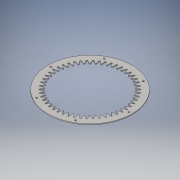
# Autodesk Inventor part: Arm Outer Gear
Saved by Autodesk Inventor 2016 (Build 200138000, 138)
## iProperties
Created: 2016-04-16
Part Number: Arm Outer Gear
Material: Generic
Document SubType Name: Modeling
Designer: rmarkowi
Density: 1 g/cm^3
Appearance: Default
Author: rmarkowi
Autodesk Inventor part; units mm, degrees
(part 1 of 2)
ref_plane "YZ Plane" through (0, 0, 0) normal (1, 0, 0) x (0, 1, 0)
ref_plane "XZ Plane" through (0, 0, 0) normal (0, 1, 0) x (-1, 0, 0)
ref_plane "XY Plane" through (0, 0, 0) normal (0, 0, 1) x (1, 0, 0)
sketch "Sketch1" plane through (0, 0, 0) normal (0, 1, 0) x (-1, 0, 0)
  circle A0 centre (0, 0) radius 120.65 construction
  line L0 (0, 0) -> (120.65, 0) construction
  line L1 (120.65, 120.65) -> (120.65, -120.65) construction
  line L2 (79.3853, 113.3739) -> (161.9147, -113.3739) construction
  line L3 (106.5438, 38.7788) -> (0, 0) construction
  arc A1 (106.5438, 38.7788) -> (102.7586, 47.9171) centre (0, 0) ccw construction
  line L4 (0, 0) -> (102.7586, 47.9171) construction
  line L5 (0, 0) -> (106.5438, 38.7788) construction
  line L6 (102.7586, 47.9171) -> (126.968, 2.8527) construction
  arc A2 (110.9039, 23.5734) -> (106.5438, 38.7788) centre (0, 0) ccw construction
  line L7 (0, 0) -> (110.9039, 23.5734) construction
  line L8 (0, 0) -> (106.5438, 38.7788) construction
  line L9 (110.9039, 23.5734) -> (116.206, -1.371) construction
  line L10 (115.9739, -1.4203) -> (113.3644, -1.975) construction
  spline S0 degree 3 poles (125.457, 2.1829) (119.9346, -0.2189) (115.9739, -1.4203) (113.3644, -1.975) knots 1.081688 1.081688 1.081688 1.081688 2 2 2 2
  line L11 (0, 0) -> (153.1146, 4.8118) construction
  line L12 (0, 0) -> (153.1902, 0) construction
  line L13 (0, 0) -> (153.1146, -4.8118) construction
  line L14 (115.8342, -5.8646) -> (113.2647, -5.1471) construction
  spline S1 degree 3 poles (125.0724, -10.0561) (119.7117, -7.3123) (115.8342, -5.8646) (113.2647, -5.1471) knots 1.081688 1.081688 1.081688 1.081688 2 2 2 2
  circle A3 centre (0, 0) radius 125.476 construction
  line L15 (125.457, 2.1829) -> (119.9346, -0.2189) construction
  line L16 (119.9346, -0.2189) -> (115.9739, -1.4203) construction
  line L17 (125.0724, -10.0561) -> (119.7117, -7.3123) construction
  line L18 (119.7117, -7.3123) -> (115.8342, -5.8646) construction
  arc A4 (126.6012, -10.0561) -> (126.9812, 2.1829) centre (0, 0) ccw
  arc A5 (113.2647, -5.1471) -> (113.3644, -1.975) centre (0, 0) ccw
  line L19 (125.457, 2.1829) -> (126.9812, 2.1829)
  line L20 (125.0724, -10.0561) -> (126.6012, -10.0561)
  arc A6 (113.0167, 9.0893) -> (112.718, 12.2489) centre (0, 0) ccw
  line L21 (115.6558, 8.6996) -> (113.0167, 9.0893) construction
  spline S2 degree 3 poles (124.1942, 17.8896) (119.0164, 14.8147) (115.2374, 13.1263) (112.718, 12.2489) knots 1.081688 1.081688 1.081688 1.081688 2 2 2 2
  line L22 (124.1942, 17.8896) -> (119.0164, 14.8147) construction
  line L23 (119.0164, 14.8147) -> (115.2374, 13.1263) construction
  line L24 (115.2374, 13.1263) -> (112.718, 12.2489) construction
  spline S3 degree 3 poles (125.3465, 5.6989) (119.6842, 7.7492) (115.6558, 8.6996) (113.0167, 9.0893) knots 1.081688 1.081688 1.081688 1.081688 2 2 2 2
  line L25 (125.3465, 5.6989) -> (119.6842, 7.7492) construction
  line L26 (119.6842, 7.7492) -> (115.6558, 8.6996) construction
  arc A7 (126.8633, 5.8906) -> (125.7064, 18.0806) centre (0, 0) ccw
  line L27 (125.3465, 5.6989) -> (126.8633, 5.8906)
  line L28 (124.1942, 17.8896) -> (125.7064, 18.0806)
  arc A8 (110.9863, 23.1824) -> (110.294, 26.2796) centre (0, 0) ccw
  line L29 (113.6535, 23.1265) -> (110.9863, 23.1824) construction
  spline S4 degree 3 poles (120.9727, 33.3142) (116.2211, 29.6145) (112.6836, 27.4658) (110.294, 26.2796) knots 1.081688 1.081688 1.081688 1.081688 2 2 2 2
  line L30 (120.9727, 33.3142) -> (116.2211, 29.6145) construction
  line L31 (116.2211, 29.6145) -> (112.6836, 27.4658) construction
  line L32 (112.6836, 27.4658) -> (110.294, 26.2796) construction
  spline S5 degree 3 poles (123.6439, 21.3641) (117.7693, 22.6885) (113.6535, 23.1265) (110.9863, 23.1824) knots 1.081688 1.081688 1.081688 1.081688 2 2 2 2
  line L33 (123.6439, 21.3641) -> (117.7693, 22.6885) construction
  line L34 (117.7693, 22.6885) -> (113.6535, 23.1265) construction
  arc A9 (125.1247, 21.7443) -> (122.449, 33.6932) centre (0, 0) ccw
  line L35 (123.6439, 21.3641) -> (125.1247, 21.7443)
  line L36 (120.9727, 33.3142) -> (122.449, 33.6932)
  arc A10 (107.2056, 36.9098) -> (106.1306, 39.8959) centre (0, 0) ccw
  line L37 (109.8588, 37.1887) -> (107.2056, 36.9098) construction
  spline S6 degree 3 poles (115.8434, 48.2134) (111.593, 43.9474) (108.3526, 41.3723) (106.1306, 39.8959) knots 1.081688 1.081688 1.081688 1.081688 2 2 2 2
  line L38 (115.8434, 48.2134) -> (111.593, 43.9474) construction
  line L39 (111.593, 43.9474) -> (108.3526, 41.3723) construction
  line L40 (108.3526, 41.3723) -> (106.1306, 39.8959) construction
  spline S7 degree 3 poles (119.9913, 36.6923) (113.997, 37.27) (109.8588, 37.1887) (107.2056, 36.9098) knots 1.081688 1.081688 1.081688 1.081688 2 2 2 2
  line L41 (119.9913, 36.6923) -> (113.997, 37.27) construction
  line L42 (113.997, 37.27) -> (109.8588, 37.1887) construction
  arc A11 (121.4127, 37.2551) -> (117.2606, 48.7745) centre (0, 0) ccw
  line L43 (119.9913, 36.6923) -> (121.4127, 37.2551)
  line L44 (115.8434, 48.2134) -> (117.2606, 48.7745)
  arc A12 (101.7343, 50.0552) -> (100.2934, 52.883) centre (0, 0) ccw
  line L45 (104.3316, 50.6644) -> (101.7343, 50.0552) construction
  spline S8 degree 3 poles (108.8872, 62.3522) (105.205, 57.5872) (102.3129, 54.6262) (100.2934, 52.883) knots 1.081688 1.081688 1.081688 1.081688 2 2 2 2
  line L46 (108.8872, 62.3522) -> (105.205, 57.5872) construction
  line L47 (105.205, 57.5872) -> (102.3129, 54.6262) construction
  line L48 (102.3129, 54.6262) -> (100.2934, 52.883) construction
  spline S9 degree 3 poles (114.4463, 51.4419) (108.4269, 51.2637) (104.3316, 50.6644) (101.7343, 50.0552) knots 1.081688 1.081688 1.081688 1.081688 2 2 2 2
  line L49 (114.4463, 51.4419) -> (108.4269, 51.2637) construction
  line L50 (108.4269, 51.2637) -> (104.3316, 50.6644) construction
  arc A13 (115.7861, 52.1784) -> (110.2229, 63.0865) centre (0, 0) ccw
  line L51 (114.4463, 51.4419) -> (115.7861, 52.1784)
  line L52 (108.8872, 62.3522) -> (110.2229, 63.0865)
  arc A14 (94.6585, 62.4112) -> (92.8746, 65.0361) centre (0, 0) ccw
  line L53 (97.1589, 63.3411) -> (94.6585, 62.4112) construction
  spline S10 degree 3 poles (100.2138, 75.5078) (97.1578, 70.3187) (94.6597, 67.0187) (92.8746, 65.0361) knots 1.081688 1.081688 1.081688 1.081688 2 2 2 2
  line L54 (100.2138, 75.5078) -> (97.1578, 70.3187) construction
  line L55 (97.1578, 70.3187) -> (94.6597, 67.0187) construction
  line L56 (94.6597, 67.0187) -> (92.8746, 65.0361) construction
  spline S11 degree 3 poles (107.0965, 65.3802) (101.1469, 64.449) (97.1589, 63.3411) (94.6585, 62.4112) knots 1.081688 1.081688 1.081688 1.081688 2 2 2 2
  line L57 (107.0965, 65.3802) -> (101.1469, 64.449) construction
  line L58 (101.1469, 64.449) -> (97.1589, 63.3411) construction
  arc A15 (108.3334, 66.2788) -> (101.4469, 76.4037) centre (0, 0) ccw
  line L59 (107.0965, 65.3802) -> (108.3334, 66.2788)
  line L60 (100.2138, 75.5078) -> (101.4469, 76.4037)
  arc A16 (86.0899, 73.7829) -> (83.991, 76.1636) centre (0, 0) ccw
  line L61 (88.4541, 75.0189) -> (86.0899, 73.7829) construction
  spline S12 degree 3 poles (89.9599, 87.4725) (87.5784, 81.9414) (85.5136, 78.3542) (83.991, 76.1636) knots 1.081688 1.081688 1.081688 1.081688 2 2 2 2
  line L62 (89.9599, 87.4725) -> (87.5784, 81.9414) construction
  line L63 (87.5784, 81.9414) -> (85.5136, 78.3542) construction
  line L64 (85.5136, 78.3542) -> (83.991, 76.1636) construction
  spline S13 degree 3 poles (98.0577, 78.2874) (92.2717, 76.6179) (88.4541, 75.0189) (86.0899, 73.7829) knots 1.081688 1.081688 1.081688 1.081688 2 2 2 2
  line L65 (98.0577, 78.2874) -> (92.2717, 76.6179) construction
  line L66 (92.2717, 76.6179) -> (88.4541, 75.0189) construction
  arc A17 (99.1722, 79.334) -> (91.0711, 88.5159) centre (0, 0) ccw
  line L67 (98.0577, 78.2874) -> (99.1722, 79.334)
  line L68 (89.9599, 87.4725) -> (91.0711, 88.5159)
  arc A18 (76.1636, 83.991) -> (73.7829, 86.0899) centre (0, 0) ccw
  line L69 (78.3542, 85.5136) -> (76.1636, 83.991) construction
  spline S14 degree 3 poles (78.2874, 98.0577) (76.6179, 92.2717) (75.0189, 88.4541) (73.7829, 86.0899) knots 1.081688 1.081688 1.081688 1.081688 2 2 2 2
  line L70 (78.2874, 98.0577) -> (76.6179, 92.2717) construction
  line L71 (76.6179, 92.2717) -> (75.0189, 88.4541) construction
  line L72 (75.0189, 88.4541) -> (73.7829, 86.0899) construction
  spline S15 degree 3 poles (87.4725, 89.9599) (81.9414, 87.5784) (78.3542, 85.5136) (76.1636, 83.991) knots 1.081688 1.081688 1.081688 1.081688 2 2 2 2
  line L73 (87.4725, 89.9599) -> (81.9414, 87.5784) construction
  line L74 (81.9414, 87.5784) -> (78.3542, 85.5136) construction
  arc A19 (88.447, 91.138) -> (79.259, 99.2321) centre (0, 0) ccw
  line L75 (87.4725, 89.9599) -> (88.447, 91.138)
  line L76 (78.2874, 98.0577) -> (79.259, 99.2321)
  arc A20 (65.0361, 92.8746) -> (62.4112, 94.6585) centre (0, 0) ccw
  line L77 (67.0187, 94.6597) -> (65.0361, 92.8746) construction
  spline S16 degree 3 poles (65.3802, 107.0965) (64.449, 101.1469) (63.3411, 97.1589) (62.4112, 94.6585) knots 1.081688 1.081688 1.081688 1.081688 2 2 2 2
  line L78 (65.3802, 107.0965) -> (64.449, 101.1469) construction
  line L79 (64.449, 101.1469) -> (63.3411, 97.1589) construction
  line L80 (63.3411, 97.1589) -> (62.4112, 94.6585) construction
  spline S17 degree 3 poles (75.5078, 100.2138) (70.3187, 97.1578) (67.0187, 94.6597) (65.0361, 92.8746) knots 1.081688 1.081688 1.081688 1.081688 2 2 2 2
  line L81 (75.5078, 100.2138) -> (70.3187, 97.1578) construction
  line L82 (70.3187, 97.1578) -> (67.0187, 94.6597) construction
  arc A21 (76.327, 101.5047) -> (66.1969, 108.3834) centre (0, 0) ccw
  line L83 (75.5078, 100.2138) -> (76.327, 101.5047)
  line L84 (65.3802, 107.0965) -> (66.1969, 108.3834)
  arc A22 (52.883, 100.2934) -> (50.0552, 101.7343) centre (0, 0) ccw
  line L85 (54.6262, 102.3129) -> (52.883, 100.2934) construction
  spline S18 degree 3 poles (51.4419, 114.4463) (51.2637, 108.4269) (50.6644, 104.3316) (50.0552, 101.7343) knots 1.081688 1.081688 1.081688 1.081688 2 2 2 2
  line L86 (51.4419, 114.4463) -> (51.2637, 108.4269) construction
  line L87 (51.2637, 108.4269) -> (50.6644, 104.3316) construction
  line L88 (50.6644, 104.3316) -> (50.0552, 101.7343) construction
  spline S19 degree 3 poles (62.3522, 108.8872) (57.5872, 105.205) (54.6262, 102.3129) (52.883, 100.2934) knots 1.081688 1.081688 1.081688 1.081688 2 2 2 2
  line L89 (62.3522, 108.8872) -> (57.5872, 105.205) construction
  line L90 (57.5872, 105.205) -> (54.6262, 102.3129) construction
  arc A23 (63.0032, 110.2706) -> (52.0909, 115.8255) centre (0, 0) ccw
  line L91 (62.3522, 108.8872) -> (63.0032, 110.2706)
  line L92 (51.4419, 114.4463) -> (52.0909, 115.8255)
  arc A24 (39.8959, 106.1306) -> (36.9098, 107.2056) centre (0, 0) ccw
  line L93 (41.3723, 108.3526) -> (39.8959, 106.1306) construction
  spline S20 degree 3 poles (36.6923, 119.9913) (37.27, 113.997) (37.1887, 109.8588) (36.9098, 107.2056) knots 1.081688 1.081688 1.081688 1.081688 2 2 2 2
  line L94 (36.6923, 119.9913) -> (37.27, 113.997) construction
  line L95 (37.27, 113.997) -> (37.1887, 109.8588) construction
  line L96 (37.1887, 109.8588) -> (36.9098, 107.2056) construction
  spline S21 degree 3 poles (48.2134, 115.8434) (43.9474, 111.593) (41.3723, 108.3526) (39.8959, 106.1306) knots 1.081688 1.081688 1.081688 1.081688 2 2 2 2
  line L97 (48.2134, 115.8434) -> (43.9474, 111.593) construction
  line L98 (43.9474, 111.593) -> (41.3723, 108.3526) construction
  arc A25 (48.6858, 117.2974) -> (37.1633, 121.4409) centre (0, 0) ccw
  line L99 (48.2134, 115.8434) -> (48.6858, 117.2974)
  line L100 (36.6923, 119.9913) -> (37.1633, 121.4409)
  arc A26 (26.2796, 110.294) -> (23.1824, 110.9863) centre (0, 0) ccw
  line L101 (27.4658, 112.6836) -> (26.2796, 110.294) construction
  spline S22 degree 3 poles (21.3641, 123.6439) (22.6885, 117.7693) (23.1265, 113.6535) (23.1824, 110.9863) knots 1.081688 1.081688 1.081688 1.081688 2 2 2 2
  line L102 (21.3641, 123.6439) -> (22.6885, 117.7693) construction
  line L103 (22.6885, 117.7693) -> (23.1265, 113.6535) construction
  line L104 (23.1265, 113.6535) -> (23.1824, 110.9863) construction
  spline S23 degree 3 poles (33.3142, 120.9727) (29.6145, 116.2211) (27.4658, 112.6836) (26.2796, 110.294) knots 1.081688 1.081688 1.081688 1.081688 2 2 2 2
  line L105 (33.3142, 120.9727) -> (29.6145, 116.2211) construction
  line L106 (29.6145, 116.2211) -> (27.4658, 112.6836) construction
  arc A27 (33.6007, 122.4745) -> (21.6497, 125.1411) centre (0, 0) ccw
  line L107 (33.3142, 120.9727) -> (33.6007, 122.4745)
  line L108 (21.3641, 123.6439) -> (21.6497, 125.1411)
  arc A28 (12.2489, 112.718) -> (9.0893, 113.0167) centre (0, 0) ccw
  line L109 (13.1263, 115.2374) -> (12.2489, 112.718) construction
  spline S24 degree 3 poles (5.6989, 125.3465) (7.7492, 119.6842) (8.6996, 115.6558) (9.0893, 113.0167) knots 1.081688 1.081688 1.081688 1.081688 2 2 2 2
  line L110 (5.6989, 125.3465) -> (7.7492, 119.6842) construction
  line L111 (7.7492, 119.6842) -> (8.6996, 115.6558) construction
  line L112 (8.6996, 115.6558) -> (9.0893, 113.0167) construction
  spline S25 degree 3 poles (17.8896, 124.1942) (14.8147, 119.0164) (13.1263, 115.2374) (12.2489, 112.718) knots 1.081688 1.081688 1.081688 1.081688 2 2 2 2
  line L113 (17.8896, 124.1942) -> (14.8147, 119.0164) construction
  line L114 (14.8147, 119.0164) -> (13.1263, 115.2374) construction
  arc A29 (17.9856, 125.72) -> (5.7947, 126.8677) centre (0, 0) ccw
  line L115 (17.8896, 124.1942) -> (17.9856, 125.72)
  line L116 (5.6989, 125.3465) -> (5.7947, 126.8677)
  arc A30 (-1.975, 113.3644) -> (-5.1471, 113.2647) centre (0, 0) ccw
  line L117 (-1.4203, 115.9739) -> (-1.975, 113.3644) construction
  spline S26 degree 3 poles (-10.0561, 125.0724) (-7.3123, 119.7117) (-5.8646, 115.8342) (-5.1471, 113.2647) knots 1.081688 1.081688 1.081688 1.081688 2 2 2 2
  line L118 (-10.0561, 125.0724) -> (-7.3123, 119.7117) construction
  line L119 (-7.3123, 119.7117) -> (-5.8646, 115.8342) construction
  line L120 (-5.8646, 115.8342) -> (-5.1471, 113.2647) construction
  spline S27 degree 3 poles (2.1829, 125.457) (-0.2189, 119.9346) (-1.4203, 115.9739) (-1.975, 113.3644) knots 1.081688 1.081688 1.081688 1.081688 2 2 2 2
  line L121 (2.1829, 125.457) -> (-0.2189, 119.9346) construction
  line L122 (-0.2189, 119.9346) -> (-1.4203, 115.9739) construction
  arc A31 (2.0869, 126.9829) -> (-10.1518, 126.5936) centre (0, 0) ccw
  line L123 (2.1829, 125.457) -> (2.0869, 126.9829)
  line L124 (-10.0561, 125.0724) -> (-10.1518, 126.5936)
  arc A32 (-16.1677, 112.2229) -> (-19.3024, 111.7265) centre (0, 0) ccw
  line L125 (-15.9445, 114.8814) -> (-16.1677, 112.2229) construction
  spline S28 degree 3 poles (-25.6525, 122.8258) (-22.2585, 117.8513) (-20.3362, 114.1858) (-19.3024, 111.7265) knots 1.081688 1.081688 1.081688 1.081688 2 2 2 2
  line L126 (-25.6525, 122.8258) -> (-22.2585, 117.8513) construction
  line L127 (-22.2585, 117.8513) -> (-20.3362, 114.1858) construction
  line L128 (-20.3362, 114.1858) -> (-19.3024, 111.7265) construction
  spline S29 degree 3 poles (-13.5583, 124.7413) (-15.2489, 118.9615) (-15.9445, 114.8814) (-16.1677, 112.2229) knots 1.081688 1.081688 1.081688 1.081688 2 2 2 2
  line L129 (-13.5583, 124.7413) -> (-15.2489, 118.9615) construction
  line L130 (-15.2489, 118.9615) -> (-15.9445, 114.8814) construction
  arc A33 (-13.8448, 126.2431) -> (-25.9381, 124.323) centre (0, 0) ccw
  line L131 (-13.5583, 124.7413) -> (-13.8448, 126.2431)
  line L132 (-25.6525, 122.8258) -> (-25.9381, 124.323)
  arc A34 (-30.1055, 109.3117) -> (-33.1532, 108.4262) centre (0, 0) ccw
  line L133 (-30.2172, 111.9771) -> (-30.1055, 109.3117) construction
  spline S30 degree 3 poles (-40.8444, 118.6422) (-36.8537, 114.1323) (-34.4871, 110.7366) (-33.1532, 108.4262) knots 1.081688 1.081688 1.081688 1.081688 2 2 2 2
  line L134 (-40.8444, 118.6422) -> (-36.8537, 114.1323) construction
  line L135 (-36.8537, 114.1323) -> (-34.4871, 110.7366) construction
  line L136 (-34.4871, 110.7366) -> (-33.1532, 108.4262) construction
  spline S31 degree 3 poles (-29.0856, 122.0584) (-30.0385, 116.1122) (-30.2172, 111.9771) (-30.1055, 109.3117) knots 1.081688 1.081688 1.081688 1.081688 2 2 2 2
  line L137 (-29.0856, 122.0584) -> (-30.0385, 116.1122) construction
  line L138 (-30.0385, 116.1122) -> (-30.2172, 111.9771) construction
  arc A35 (-29.558, 123.5124) -> (-41.3154, 120.0918) centre (0, 0) ccw
  line L139 (-29.0856, 122.0584) -> (-29.558, 123.5124)
  line L140 (-40.8444, 118.6422) -> (-41.3154, 120.0918)
  arc A36 (-43.5685, 104.6765) -> (-46.4812, 103.4161) centre (0, 0) ccw
  line L141 (-44.0134, 107.3069) -> (-43.5685, 104.6765) construction
  spline S32 degree 3 poles (-55.3921, 112.5875) (-50.8677, 108.6133) (-48.0941, 105.541) (-46.4812, 103.4161) knots 1.081688 1.081688 1.081688 1.081688 2 2 2 2
  line L142 (-55.3921, 112.5875) -> (-50.8677, 108.6133) construction
  line L143 (-50.8677, 108.6133) -> (-48.0941, 105.541) construction
  line L144 (-48.0941, 105.541) -> (-46.4812, 103.4161) construction
  spline S33 degree 3 poles (-44.1542, 117.4505) (-44.3544, 111.4318) (-44.0134, 107.3069) (-43.5685, 104.6765) knots 1.081688 1.081688 1.081688 1.081688 2 2 2 2
  line L145 (-44.1542, 117.4505) -> (-44.3544, 111.4318) construction
  line L146 (-44.3544, 111.4318) -> (-44.0134, 107.3069) construction
  arc A37 (-44.8052, 118.8339) -> (-56.0411, 113.9666) centre (0, 0) ccw
  line L147 (-44.1542, 117.4505) -> (-44.8052, 118.8339)
  line L148 (-55.3921, 112.5875) -> (-56.0411, 113.9666)
  arc A38 (-56.3444, 98.3905) -> (-59.0761, 96.775) centre (0, 0) ccw
  line L149 (-57.1155, 100.9444) -> (-56.3444, 98.3905) construction
  spline S34 degree 3 poles (-69.0663, 104.7572) (-64.0794, 101.3814) (-60.9427, 98.681) (-59.0761, 96.775) knots 1.081688 1.081688 1.081688 1.081688 2 2 2 2
  line L150 (-69.0663, 104.7572) -> (-64.0794, 101.3814) construction
  line L151 (-64.0794, 101.3814) -> (-60.9427, 98.681) construction
  line L152 (-60.9427, 98.681) -> (-59.0761, 96.775) construction
  spline S35 degree 3 poles (-58.5265, 110.9904) (-57.9708, 104.9941) (-57.1155, 100.9444) (-56.3444, 98.3905) knots 1.081688 1.081688 1.081688 1.081688 2 2 2 2
  line L153 (-58.5265, 110.9904) -> (-57.9708, 104.9941) construction
  line L154 (-57.9708, 104.9941) -> (-57.1155, 100.9444) construction
  arc A39 (-59.3457, 112.2813) -> (-69.883, 106.0442) centre (0, 0) ccw
  line L155 (-58.5265, 110.9904) -> (-59.3457, 112.2813)
  line L156 (-69.0663, 104.7572) -> (-69.883, 106.0442)
  arc A40 (-68.2317, 90.5528) -> (-70.7394, 88.6077) centre (0, 0) ccw
  line L157 (-69.3168, 92.99) -> (-68.2317, 90.5528) construction
  spline S36 degree 3 poles (-81.6512, 95.2749) (-76.2806, 92.5507) (-72.8302, 90.2647) (-70.7394, 88.6077) knots 1.081688 1.081688 1.081688 1.081688 2 2 2 2
  line L158 (-81.6512, 95.2749) -> (-76.2806, 92.5507) construction
  line L159 (-76.2806, 92.5507) -> (-72.8302, 90.2647) construction
  line L160 (-72.8302, 90.2647) -> (-70.7394, 88.6077) construction
  spline S37 degree 3 poles (-71.9758, 102.7799) (-70.6729, 96.9005) (-69.3168, 92.99) (-68.2317, 90.5528) knots 1.081688 1.081688 1.081688 1.081688 2 2 2 2
  line L161 (-71.9758, 102.7799) -> (-70.6729, 96.9005) construction
  line L162 (-70.6729, 96.9005) -> (-69.3168, 92.99) construction
  arc A41 (-72.9503, 103.9579) -> (-82.6228, 96.4493) centre (0, 0) ccw
  line L163 (-71.9758, 102.7799) -> (-72.9503, 103.9579)
  line L164 (-81.6512, 95.2749) -> (-82.6228, 96.4493)
  arc A42 (-79.043, 81.2871) -> (-81.2871, 79.043) centre (0, 0) ccw
  line L165 (-80.4249, 83.569) -> (-79.043, 81.2871) construction
  spline S38 degree 3 poles (-92.9485, 84.29) (-87.2788, 82.2605) (-83.569, 80.4249) (-81.2871, 79.043) knots 1.081688 1.081688 1.081688 1.081688 2 2 2 2
  line L166 (-92.9485, 84.29) -> (-87.2788, 82.2605) construction
  line L167 (-87.2788, 82.2605) -> (-83.569, 80.4249) construction
  line L168 (-83.569, 80.4249) -> (-81.2871, 79.043) construction
  spline S39 degree 3 poles (-84.29, 92.9485) (-82.2605, 87.2788) (-80.4249, 83.569) (-79.043, 81.2871) knots 1.081688 1.081688 1.081688 1.081688 2 2 2 2
  line L169 (-84.29, 92.9485) -> (-82.2605, 87.2788) construction
  line L170 (-82.2605, 87.2788) -> (-80.4249, 83.569) construction
  arc A43 (-85.4045, 93.9951) -> (-94.0596, 85.3334) centre (0, 0) ccw
  line L171 (-84.29, 92.9485) -> (-85.4045, 93.9951)
  line L172 (-92.9485, 84.29) -> (-94.0596, 85.3334)
  arc A44 (-88.6077, 70.7394) -> (-90.5528, 68.2317) centre (0, 0) ccw
  line L173 (-90.2647, 72.8302) -> (-88.6077, 70.7394) construction
  spline S40 degree 3 poles (-102.7799, 71.9758) (-96.9005, 70.6729) (-92.99, 69.3168) (-90.5528, 68.2317) knots 1.081688 1.081688 1.081688 1.081688 2 2 2 2
  line L174 (-102.7799, 71.9758) -> (-96.9005, 70.6729) construction
  line L175 (-96.9005, 70.6729) -> (-92.99, 69.3168) construction
  line L176 (-92.99, 69.3168) -> (-90.5528, 68.2317) construction
  spline S41 degree 3 poles (-95.2749, 81.6512) (-92.5507, 76.2806) (-90.2647, 72.8302) (-88.6077, 70.7394) knots 1.081688 1.081688 1.081688 1.081688 2 2 2 2
  line L177 (-95.2749, 81.6512) -> (-92.5507, 76.2806) construction
  line L178 (-92.5507, 76.2806) -> (-90.2647, 72.8302) construction
  arc A45 (-96.5117, 82.5499) -> (-104.013, 72.8717) centre (0, 0) ccw
  line L179 (-95.2749, 81.6512) -> (-96.5117, 82.5499)
  line L180 (-102.7799, 71.9758) -> (-104.013, 72.8717)
  arc A46 (-96.775, 59.0761) -> (-98.3905, 56.3444) centre (0, 0) ccw
  line L181 (-98.681, 60.9427) -> (-96.775, 59.0761) construction
  spline S42 degree 3 poles (-110.9904, 58.5265) (-104.9941, 57.9708) (-100.9444, 57.1155) (-98.3905, 56.3444) knots 1.081688 1.081688 1.081688 1.081688 2 2 2 2
  line L182 (-110.9904, 58.5265) -> (-104.9941, 57.9708) construction
  line L183 (-104.9941, 57.9708) -> (-100.9444, 57.1155) construction
  line L184 (-100.9444, 57.1155) -> (-98.3905, 56.3444) construction
  spline S43 degree 3 poles (-104.7572, 69.0663) (-101.3814, 64.0794) (-98.681, 60.9427) (-96.775, 59.0761) knots 1.081688 1.081688 1.081688 1.081688 2 2 2 2
  line L185 (-104.7572, 69.0663) -> (-101.3814, 64.0794) construction
  line L186 (-101.3814, 64.0794) -> (-98.681, 60.9427) construction
  arc A47 (-106.097, 69.8028) -> (-112.3261, 59.2608) centre (0, 0) ccw
  line L187 (-104.7572, 69.0663) -> (-106.097, 69.8028)
  line L188 (-110.9904, 58.5265) -> (-112.3261, 59.2608)
  arc A48 (-103.4161, 46.4812) -> (-104.6765, 43.5685) centre (0, 0) ccw
  line L189 (-105.541, 48.0941) -> (-103.4161, 46.4812) construction
  spline S44 degree 3 poles (-117.4505, 44.1542) (-111.4318, 44.3544) (-107.3069, 44.0134) (-104.6765, 43.5685) knots 1.081688 1.081688 1.081688 1.081688 2 2 2 2
  line L190 (-117.4505, 44.1542) -> (-111.4318, 44.3544) construction
  line L191 (-111.4318, 44.3544) -> (-107.3069, 44.0134) construction
  line L192 (-107.3069, 44.0134) -> (-104.6765, 43.5685) construction
  spline S45 degree 3 poles (-112.5875, 55.3921) (-108.6133, 50.8677) (-105.541, 48.0941) (-103.4161, 46.4812) knots 1.081688 1.081688 1.081688 1.081688 2 2 2 2
  line L193 (-112.5875, 55.3921) -> (-108.6133, 50.8677) construction
  line L194 (-108.6133, 50.8677) -> (-105.541, 48.0941) construction
  arc A49 (-114.009, 55.9549) -> (-118.8677, 44.7153) centre (0, 0) ccw
  line L195 (-112.5875, 55.3921) -> (-114.009, 55.9549)
  line L196 (-117.4505, 44.1542) -> (-118.8677, 44.7153)
  arc A50 (-108.4262, 33.1532) -> (-109.3117, 30.1055) centre (0, 0) ccw
  line L197 (-110.7366, 34.4871) -> (-108.4262, 33.1532) construction
  spline S46 degree 3 poles (-122.0584, 29.0856) (-116.1122, 30.0385) (-111.9771, 30.2172) (-109.3117, 30.1055) knots 1.081688 1.081688 1.081688 1.081688 2 2 2 2
  line L198 (-122.0584, 29.0856) -> (-116.1122, 30.0385) construction
  line L199 (-116.1122, 30.0385) -> (-111.9771, 30.2172) construction
  line L200 (-111.9771, 30.2172) -> (-109.3117, 30.1055) construction
  spline S47 degree 3 poles (-118.6422, 40.8444) (-114.1323, 36.8537) (-110.7366, 34.4871) (-108.4262, 33.1532) knots 1.081688 1.081688 1.081688 1.081688 2 2 2 2
  line L201 (-118.6422, 40.8444) -> (-114.1323, 36.8537) construction
  line L202 (-114.1323, 36.8537) -> (-110.7366, 34.4871) construction
  arc A51 (-120.123, 41.2246) -> (-123.5347, 29.4647) centre (0, 0) ccw
  line L203 (-118.6422, 40.8444) -> (-120.123, 41.2246)
  line L204 (-122.0584, 29.0856) -> (-123.5347, 29.4647)
  arc A52 (-111.7265, 19.3024) -> (-112.2229, 16.1677) centre (0, 0) ccw
  line L205 (-114.1858, 20.3362) -> (-111.7265, 19.3024) construction
  spline S48 degree 3 poles (-124.7413, 13.5583) (-118.9615, 15.2489) (-114.8814, 15.9445) (-112.2229, 16.1677) knots 1.081688 1.081688 1.081688 1.081688 2 2 2 2
  line L206 (-124.7413, 13.5583) -> (-118.9615, 15.2489) construction
  line L207 (-118.9615, 15.2489) -> (-114.8814, 15.9445) construction
  line L208 (-114.8814, 15.9445) -> (-112.2229, 16.1677) construction
  spline S49 degree 3 poles (-122.8258, 25.6525) (-117.8513, 22.2585) (-114.1858, 20.3362) (-111.7265, 19.3024) knots 1.081688 1.081688 1.081688 1.081688 2 2 2 2
  line L209 (-122.8258, 25.6525) -> (-117.8513, 22.2585) construction
  line L210 (-117.8513, 22.2585) -> (-114.1858, 20.3362) construction
  arc A53 (-124.3426, 25.8441) -> (-126.2535, 13.7493) centre (0, 0) ccw
  line L211 (-122.8258, 25.6525) -> (-124.3426, 25.8441)
  line L212 (-124.7413, 13.5583) -> (-126.2535, 13.7493)
  arc A54 (-113.2647, 5.1471) -> (-113.3644, 1.975) centre (0, 0) ccw
  line L213 (-115.8342, 5.8646) -> (-113.2647, 5.1471) construction
  spline S50 degree 3 poles (-125.457, -2.1829) (-119.9346, 0.2189) (-115.9739, 1.4203) (-113.3644, 1.975) knots 1.081688 1.081688 1.081688 1.081688 2 2 2 2
  line L214 (-125.457, -2.1829) -> (-119.9346, 0.2189) construction
  line L215 (-119.9346, 0.2189) -> (-115.9739, 1.4203) construction
  line L216 (-115.9739, 1.4203) -> (-113.3644, 1.975) construction
  spline S51 degree 3 poles (-125.0724, 10.0561) (-119.7117, 7.3123) (-115.8342, 5.8646) (-113.2647, 5.1471) knots 1.081688 1.081688 1.081688 1.081688 2 2 2 2
  line L217 (-125.0724, 10.0561) -> (-119.7117, 7.3123) construction
  line L218 (-119.7117, 7.3123) -> (-115.8342, 5.8646) construction
  arc A55 (-126.6012, 10.0561) -> (-126.9812, -2.1829) centre (0, 0) ccw
  line L219 (-125.0724, 10.0561) -> (-126.6012, 10.0561)
  line L220 (-125.457, -2.1829) -> (-126.9812, -2.1829)
  arc A56 (-113.0167, -9.0893) -> (-112.718, -12.2489) centre (0, 0) ccw
  line L221 (-115.6558, -8.6996) -> (-113.0167, -9.0893) construction
  spline S52 degree 3 poles (-124.1942, -17.8896) (-119.0164, -14.8147) (-115.2374, -13.1263) (-112.718, -12.2489) knots 1.081688 1.081688 1.081688 1.081688 2 2 2 2
  line L222 (-124.1942, -17.8896) -> (-119.0164, -14.8147) construction
  line L223 (-119.0164, -14.8147) -> (-115.2374, -13.1263) construction
  line L224 (-115.2374, -13.1263) -> (-112.718, -12.2489) construction
  spline S53 degree 3 poles (-125.3465, -5.6989) (-119.6842, -7.7492) (-115.6558, -8.6996) (-113.0167, -9.0893) knots 1.081688 1.081688 1.081688 1.081688 2 2 2 2
  line L225 (-125.3465, -5.6989) -> (-119.6842, -7.7492) construction
  line L226 (-119.6842, -7.7492) -> (-115.6558, -8.6996) construction
  arc A57 (-126.8633, -5.8906) -> (-125.7064, -18.0806) centre (0, 0) ccw
  line L227 (-125.3465, -5.6989) -> (-126.8633, -5.8906)
  line L228 (-124.1942, -17.8896) -> (-125.7064, -18.0806)
  arc A58 (-110.9863, -23.1824) -> (-110.294, -26.2796) centre (0, 0) ccw
  line L229 (-113.6535, -23.1265) -> (-110.9863, -23.1824) construction
  spline S54 degree 3 poles (-120.9727, -33.3142) (-116.2211, -29.6145) (-112.6836, -27.4658) (-110.294, -26.2796) knots 1.081688 1.081688 1.081688 1.081688 2 2 2 2
  line L230 (-120.9727, -33.3142) -> (-116.2211, -29.6145) construction
  line L231 (-116.2211, -29.6145) -> (-112.6836, -27.4658) construction
  line L232 (-112.6836, -27.4658) -> (-110.294, -26.2796) construction
  spline S55 degree 3 poles (-123.6439, -21.3641) (-117.7693, -22.6885) (-113.6535, -23.1265) (-110.9863, -23.1824) knots 1.081688 1.081688 1.081688 1.081688 2 2 2 2
  line L233 (-123.6439, -21.3641) -> (-117.7693, -22.6885) construction
  line L234 (-117.7693, -22.6885) -> (-113.6535, -23.1265) construction
  arc A59 (-125.1247, -21.7443) -> (-122.449, -33.6932) centre (0, 0) ccw
  line L235 (-123.6439, -21.3641) -> (-125.1247, -21.7443)
  line L236 (-120.9727, -33.3142) -> (-122.449, -33.6932)
  arc A60 (-107.2056, -36.9098) -> (-106.1306, -39.8959) centre (0, 0) ccw
  line L237 (-109.8588, -37.1887) -> (-107.2056, -36.9098) construction
  spline S56 degree 3 poles (-115.8434, -48.2134) (-111.593, -43.9474) (-108.3526, -41.3723) (-106.1306, -39.8959) knots 1.081688 1.081688 1.081688 1.081688 2 2 2 2
  line L238 (-115.8434, -48.2134) -> (-111.593, -43.9474) construction
  line L239 (-111.593, -43.9474) -> (-108.3526, -41.3723) construction
  line L240 (-108.3526, -41.3723) -> (-106.1306, -39.8959) construction
  spline S57 degree 3 poles (-119.9913, -36.6923) (-113.997, -37.27) (-109.8588, -37.1887) (-107.2056, -36.9098) knots 1.081688 1.081688 1.081688 1.081688 2 2 2 2
  line L241 (-119.9913, -36.6923) -> (-113.997, -37.27) construction
  line L242 (-113.997, -37.27) -> (-109.8588, -37.1887) construction
  arc A61 (-121.4127, -37.2551) -> (-117.2606, -48.7745) centre (0, 0) ccw
  line L243 (-119.9913, -36.6923) -> (-121.4127, -37.2551)
  line L244 (-115.8434, -48.2134) -> (-117.2606, -48.7745)
  arc A62 (-101.7343, -50.0552) -> (-100.2934, -52.883) centre (0, 0) ccw
  line L245 (-104.3316, -50.6644) -> (-101.7343, -50.0552) construction
  spline S58 degree 3 poles (-108.8872, -62.3522) (-105.205, -57.5872) (-102.3129, -54.6262) (-100.2934, -52.883) knots 1.081688 1.081688 1.081688 1.081688 2 2 2 2
  line L246 (-108.8872, -62.3522) -> (-105.205, -57.5872) construction
  line L247 (-105.205, -57.5872) -> (-102.3129, -54.6262) construction
  line L248 (-102.3129, -54.6262) -> (-100.2934, -52.883) construction
  spline S59 degree 3 poles (-114.4463, -51.4419) (-108.4269, -51.2637) (-104.3316, -50.6644) (-101.7343, -50.0552) knots 1.081688 1.081688 1.081688 1.081688 2 2 2 2
  line L249 (-114.4463, -51.4419) -> (-108.4269, -51.2637) construction
  line L250 (-108.4269, -51.2637) -> (-104.3316, -50.6644) construction
  arc A63 (-115.7861, -52.1784) -> (-110.2229, -63.0865) centre (0, 0) ccw
  line L251 (-114.4463, -51.4419) -> (-115.7861, -52.1784)
  line L252 (-108.8872, -62.3522) -> (-110.2229, -63.0865)
  arc A64 (-94.6585, -62.4112) -> (-92.8746, -65.0361) centre (0, 0) ccw
  line L253 (-97.1589, -63.3411) -> (-94.6585, -62.4112) construction
  spline S60 degree 3 poles (-100.2138, -75.5078) (-97.1578, -70.3187) (-94.6597, -67.0187) (-92.8746, -65.0361) knots 1.081688 1.081688 1.081688 1.081688 2 2 2 2
  line L254 (-100.2138, -75.5078) -> (-97.1578, -70.3187) construction
  line L255 (-97.1578, -70.3187) -> (-94.6597, -67.0187) construction
  line L256 (-94.6597, -67.0187) -> (-92.8746, -65.0361) construction
  spline S61 degree 3 poles (-107.0965, -65.3802) (-101.1469, -64.449) (-97.1589, -63.3411) (-94.6585, -62.4112) knots 1.081688 1.081688 1.081688 1.081688 2 2 2 2
  line L257 (-107.0965, -65.3802) -> (-101.1469, -64.449) construction
  line L258 (-101.1469, -64.449) -> (-97.1589, -63.3411) construction
  arc A65 (-108.3334, -66.2788) -> (-101.4469, -76.4037) centre (0, 0) ccw
  line L259 (-107.0965, -65.3802) -> (-108.3334, -66.2788)
  line L260 (-100.2138, -75.5078) -> (-101.4469, -76.4037)
  arc A66 (-86.0899, -73.7829) -> (-83.991, -76.1636) centre (0, 0) ccw
  line L261 (-88.4541, -75.0189) -> (-86.0899, -73.7829) construction
  spline S62 degree 3 poles (-89.9599, -87.4725) (-87.5784, -81.9414) (-85.5136, -78.3542) (-83.991, -76.1636) knots 1.081688 1.081688 1.081688 1.081688 2 2 2 2
  line L262 (-89.9599, -87.4725) -> (-87.5784, -81.9414) construction
  line L263 (-87.5784, -81.9414) -> (-85.5136, -78.3542) construction
  line L264 (-85.5136, -78.3542) -> (-83.991, -76.1636) construction
  spline S63 degree 3 poles (-98.0577, -78.2874) (-92.2717, -76.6179) (-88.4541, -75.0189) (-86.0899, -73.7829) knots 1.081688 1.081688 1.081688 1.081688 2 2 2 2
  line L265 (-98.0577, -78.2874) -> (-92.2717, -76.6179) construction
  line L266 (-92.2717, -76.6179) -> (-88.4541, -75.0189) construction
  arc A67 (-99.1722, -79.334) -> (-91.0711, -88.5159) centre (0, 0) ccw
  line L267 (-98.0577, -78.2874) -> (-99.1722, -79.334)
  line L268 (-89.9599, -87.4725) -> (-91.0711, -88.5159)
  arc A68 (-76.1636, -83.991) -> (-73.7829, -86.0899) centre (0, 0) ccw
  line L269 (-78.3542, -85.5136) -> (-76.1636, -83.991) construction
  spline S64 degree 3 poles (-78.2874, -98.0577) (-76.6179, -92.2717) (-75.0189, -88.4541) (-73.7829, -86.0899) knots 1.081688 1.081688 1.081688 1.081688 2 2 2 2
  line L270 (-78.2874, -98.0577) -> (-76.6179, -92.2717) construction
  line L271 (-76.6179, -92.2717) -> (-75.0189, -88.4541) construction
  line L272 (-75.0189, -88.4541) -> (-73.7829, -86.0899) construction
  spline S65 degree 3 poles (-87.4725, -89.9599) (-81.9414, -87.5784) (-78.3542, -85.5136) (-76.1636, -83.991) knots 1.081688 1.081688 1.081688 1.081688 2 2 2 2
  line L273 (-87.4725, -89.9599) -> (-81.9414, -87.5784) construction
  line L274 (-81.9414, -87.5784) -> (-78.3542, -85.5136) construction
  arc A69 (-88.447, -91.138) -> (-79.259, -99.2321) centre (0, 0) ccw
  line L275 (-87.4725, -89.9599) -> (-88.447, -91.138)
  line L276 (-78.2874, -98.0577) -> (-79.259, -99.2321)
  arc A70 (-65.0361, -92.8746) -> (-62.4112, -94.6585) centre (0, 0) ccw
  line L277 (-67.0187, -94.6597) -> (-65.0361, -92.8746) construction
  spline S66 degree 3 poles (-65.3802, -107.0965) (-64.449, -101.1469) (-63.3411, -97.1589) (-62.4112, -94.6585) knots 1.081688 1.081688 1.081688 1.081688 2 2 2 2
  line L278 (-65.3802, -107.0965) -> (-64.449, -101.1469) construction
  line L279 (-64.449, -101.1469) -> (-63.3411, -97.1589) construction
  line L280 (-63.3411, -97.1589) -> (-62.4112, -94.6585) construction
  spline S67 degree 3 poles (-75.5078, -100.2138) (-70.3187, -97.1578) (-67.0187, -94.6597) (-65.0361, -92.8746) knots 1.081688 1.081688 1.081688 1.081688 2 2 2 2
  line L281 (-75.5078, -100.2138) -> (-70.3187, -97.1578) construction
  line L282 (-70.3187, -97.1578) -> (-67.0187, -94.6597) construction
  arc A71 (-76.327, -101.5047) -> (-66.1969, -108.3834) centre (0, 0) ccw
  line L283 (-75.5078, -100.2138) -> (-76.327, -101.5047)
  line L284 (-65.3802, -107.0965) -> (-66.1969, -108.3834)
  arc A72 (-52.883, -100.2934) -> (-50.0552, -101.7343) centre (0, 0) ccw
  line L285 (-54.6262, -102.3129) -> (-52.883, -100.2934) construction
  spline S68 degree 3 poles (-51.4419, -114.4463) (-51.2637, -108.4269) (-50.6644, -104.3316) (-50.0552, -101.7343) knots 1.081688 1.081688 1.081688 1.081688 2 2 2 2
  line L286 (-51.4419, -114.4463) -> (-51.2637, -108.4269) construction
  line L287 (-51.2637, -108.4269) -> (-50.6644, -104.3316) construction
  line L288 (-50.6644, -104.3316) -> (-50.0552, -101.7343) construction
  spline S69 degree 3 poles (-62.3522, -108.8872) (-57.5872, -105.205) (-54.6262, -102.3129) (-52.883, -100.2934) knots 1.081688 1.081688 1.081688 1.081688 2 2 2 2
  line L289 (-62.3522, -108.8872) -> (-57.5872, -105.205) construction
  line L290 (-57.5872, -105.205) -> (-54.6262, -102.3129) construction
  arc A73 (-63.0032, -110.2706) -> (-52.0909, -115.8255) centre (0, 0) ccw
  line L291 (-62.3522, -108.8872) -> (-63.0032, -110.2706)
  line L292 (-51.4419, -114.4463) -> (-52.0909, -115.8255)
  arc A74 (-39.8959, -106.1306) -> (-36.9098, -107.2056) centre (0, 0) ccw
  line L293 (-41.3723, -108.3526) -> (-39.8959, -106.1306) construction
  spline S70 degree 3 poles (-36.6923, -119.9913) (-37.27, -113.997) (-37.1887, -109.8588) (-36.9098, -107.2056) knots 1.081688 1.081688 1.081688 1.081688 2 2 2 2
  line L294 (-36.6923, -119.9913) -> (-37.27, -113.997) construction
  line L295 (-37.27, -113.997) -> (-37.1887, -109.8588) construction
  line L296 (-37.1887, -109.8588) -> (-36.9098, -107.2056) construction
  spline S71 degree 3 poles (-48.2134, -115.8434) (-43.9474, -111.593) (-41.3723, -108.3526) (-39.8959, -106.1306) knots 1.081688 1.081688 1.081688 1.081688 2 2 2 2
  line L297 (-48.2134, -115.8434) -> (-43.9474, -111.593) construction
  line L298 (-43.9474, -111.593) -> (-41.3723, -108.3526) construction
  arc A75 (-48.6858, -117.2974) -> (-37.1633, -121.4409) centre (0, 0) ccw
  line L299 (-48.2134, -115.8434) -> (-48.6858, -117.2974)
  line L300 (-36.6923, -119.9913) -> (-37.1633, -121.4409)
  arc A76 (-26.2796, -110.294) -> (-23.1824, -110.9863) centre (0, 0) ccw
  line L301 (-27.4658, -112.6836) -> (-26.2796, -110.294) construction
  spline S72 degree 3 poles (-21.3641, -123.6439) (-22.6885, -117.7693) (-23.1265, -113.6535) (-23.1824, -110.9863) knots 1.081688 1.081688 1.081688 1.081688 2 2 2 2
  line L302 (-21.3641, -123.6439) -> (-22.6885, -117.7693) construction
  line L303 (-22.6885, -117.7693) -> (-23.1265, -113.6535) construction
  line L304 (-23.1265, -113.6535) -> (-23.1824, -110.9863) construction
  spline S73 degree 3 poles (-33.3142, -120.9727) (-29.6145, -116.2211) (-27.4658, -112.6836) (-26.2796, -110.294) knots 1.081688 1.081688 1.081688 1.081688 2 2 2 2
  line L305 (-33.3142, -120.9727) -> (-29.6145, -116.2211) construction
  line L306 (-29.6145, -116.2211) -> (-27.4658, -112.6836) construction
  arc A77 (-33.6007, -122.4745) -> (-21.6497, -125.1411) centre (0, 0) ccw
  line L307 (-33.3142, -120.9727) -> (-33.6007, -122.4745)
  line L308 (-21.3641, -123.6439) -> (-21.6497, -125.1411)
  arc A78 (-12.2489, -112.718) -> (-9.0893, -113.0167) centre (0, 0) ccw
  line L309 (-13.1263, -115.2374) -> (-12.2489, -112.718) construction
  spline S74 degree 3 poles (-5.6989, -125.3465) (-7.7492, -119.6842) (-8.6996, -115.6558) (-9.0893, -113.0167) knots 1.081688 1.081688 1.081688 1.081688 2 2 2 2
  line L310 (-5.6989, -125.3465) -> (-7.7492, -119.6842) construction
  line L311 (-7.7492, -119.6842) -> (-8.6996, -115.6558) construction
  line L312 (-8.6996, -115.6558) -> (-9.0893, -113.0167) construction
  spline S75 degree 3 poles (-17.8896, -124.1942) (-14.8147, -119.0164) (-13.1263, -115.2374) (-12.2489, -112.718) knots 1.081688 1.081688 1.081688 1.081688 2 2 2 2
  line L313 (-17.8896, -124.1942) -> (-14.8147, -119.0164) construction
  line L314 (-14.8147, -119.0164) -> (-13.1263, -115.2374) construction
  arc A79 (-17.9856, -125.72) -> (-5.7947, -126.8677) centre (0, 0) ccw
  line L315 (-17.8896, -124.1942) -> (-17.9856, -125.72)
  line L316 (-5.6989, -125.3465) -> (-5.7947, -126.8677)
  arc A80 (1.975, -113.3644) -> (5.1471, -113.2647) centre (0, 0) ccw
  line L317 (1.4203, -115.9739) -> (1.975, -113.3644) construction
  spline S76 degree 3 poles (10.0561, -125.0724) (7.3123, -119.7117) (5.8646, -115.8342) (5.1471, -113.2647) knots 1.081688 1.081688 1.081688 1.081688 2 2 2 2
  line L318 (10.0561, -125.0724) -> (7.3123, -119.7117) construction
  line L319 (7.3123, -119.7117) -> (5.8646, -115.8342) construction
  line L320 (5.8646, -115.8342) -> (5.1471, -113.2647) construction
  spline S77 degree 3 poles (-2.1829, -125.457) (0.2189, -119.9346) (1.4203, -115.9739) (1.975, -113.3644) knots 1.081688 1.081688 1.081688 1.081688 2 2 2 2
  line L321 (-2.1829, -125.457) -> (0.2189, -119.9346) construction
  line L322 (0.2189, -119.9346) -> (1.4203, -115.9739) construction
  arc A81 (-2.0869, -126.9829) -> (10.1518, -126.5936) centre (0, 0) ccw
  line L323 (-2.1829, -125.457) -> (-2.0869, -126.9829)
  line L324 (10.0561, -125.0724) -> (10.1518, -126.5936)
  arc A82 (16.1677, -112.2229) -> (19.3024, -111.7265) centre (0, 0) ccw
  line L325 (15.9445, -114.8814) -> (16.1677, -112.2229) construction
  spline S78 degree 3 poles (25.6525, -122.8258) (22.2585, -117.8513) (20.3362, -114.1858) (19.3024, -111.7265) knots 1.081688 1.081688 1.081688 1.081688 2 2 2 2
  line L326 (25.6525, -122.8258) -> (22.2585, -117.8513) construction
  line L327 (22.2585, -117.8513) -> (20.3362, -114.1858) construction
  line L328 (20.3362, -114.1858) -> (19.3024, -111.7265) construction
  spline S79 degree 3 poles (13.5583, -124.7413) (15.2489, -118.9615) (15.9445, -114.8814) (16.1677, -112.2229) knots 1.081688 1.081688 1.081688 1.081688 2 2 2 2
  line L329 (13.5583, -124.7413) -> (15.2489, -118.9615) construction
  line L330 (15.2489, -118.9615) -> (15.9445, -114.8814) construction
  arc A83 (13.8448, -126.2431) -> (25.9381, -124.323) centre (0, 0) ccw
  line L331 (13.5583, -124.7413) -> (13.8448, -126.2431)
  line L332 (25.6525, -122.8258) -> (25.9381, -124.323)
  arc A84 (30.1055, -109.3117) -> (33.1532, -108.4262) centre (0, 0) ccw
  line L333 (30.2172, -111.9771) -> (30.1055, -109.3117) construction
  spline S80 degree 3 poles (40.8444, -118.6422) (36.8537, -114.1323) (34.4871, -110.7366) (33.1532, -108.4262) knots 1.081688 1.081688 1.081688 1.081688 2 2 2 2
  line L334 (40.8444, -118.6422) -> (36.8537, -114.1323) construction
  line L335 (36.8537, -114.1323) -> (34.4871, -110.7366) construction
  line L336 (34.4871, -110.7366) -> (33.1532, -108.4262) construction
  spline S81 degree 3 poles (29.0856, -122.0584) (30.0385, -116.1122) (30.2172, -111.9771) (30.1055, -109.3117) knots 1.081688 1.081688 1.081688 1.081688 2 2 2 2
  line L337 (29.0856, -122.0584) -> (30.0385, -116.1122) construction
  line L338 (30.0385, -116.1122) -> (30.2172, -111.9771) construction
  arc A85 (29.558, -123.5124) -> (41.3154, -120.0918) centre (0, 0) ccw
  line L339 (29.0856, -122.0584) -> (29.558, -123.5124)
  line L340 (40.8444, -118.6422) -> (41.3154, -120.0918)
  arc A86 (43.5685, -104.6765) -> (46.4812, -103.4161) centre (0, 0) ccw
  line L341 (44.0134, -107.3069) -> (43.5685, -104.6765) construction
  spline S82 degree 3 poles (55.3921, -112.5875) (50.8677, -108.6133) (48.0941, -105.541) (46.4812, -103.4161) knots 1.081688 1.081688 1.081688 1.081688 2 2 2 2
  line L342 (55.3921, -112.5875) -> (50.8677, -108.6133) construction
  line L343 (50.8677, -108.6133) -> (48.0941, -105.541) construction
  line L344 (48.0941, -105.541) -> (46.4812, -103.4161) construction
  spline S83 degree 3 poles (44.1542, -117.4505) (44.3544, -111.4318) (44.0134, -107.3069) (43.5685, -104.6765) knots 1.081688 1.081688 1.081688 1.081688 2 2 2 2
  line L345 (44.1542, -117.4505) -> (44.3544, -111.4318) construction
  line L346 (44.3544, -111.4318) -> (44.0134, -107.3069) construction
  arc A87 (44.8052, -118.8339) -> (56.0411, -113.9666) centre (0, 0) ccw
  line L347 (44.1542, -117.4505) -> (44.8052, -118.8339)
  line L348 (55.3921, -112.5875) -> (56.0411, -113.9666)
  arc A88 (56.3444, -98.3905) -> (59.0761, -96.775) centre (0, 0) ccw
  line L349 (57.1155, -100.9444) -> (56.3444, -98.3905) construction
  spline S84 degree 3 poles (69.0663, -104.7572) (64.0794, -101.3814) (60.9427, -98.681) (59.0761, -96.775) knots 1.081688 1.081688 1.081688 1.081688 2 2 2 2
  line L350 (69.0663, -104.7572) -> (64.0794, -101.3814) construction
  line L351 (64.0794, -101.3814) -> (60.9427, -98.681) construction
  line L352 (60.9427, -98.681) -> (59.0761, -96.775) construction
  spline S85 degree 3 poles (58.5265, -110.9904) (57.9708, -104.9941) (57.1155, -100.9444) (56.3444, -98.3905) knots 1.081688 1.081688 1.081688 1.081688 2 2 2 2
  line L353 (58.5265, -110.9904) -> (57.9708, -104.9941) construction
  line L354 (57.9708, -104.9941) -> (57.1155, -100.9444) construction
  arc A89 (59.3457, -112.2813) -> (69.883, -106.0442) centre (0, 0) ccw
  line L355 (58.5265, -110.9904) -> (59.3457, -112.2813)
  line L356 (69.0663, -104.7572) -> (69.883, -106.0442)
  arc A90 (68.2317, -90.5528) -> (70.7394, -88.6077) centre (0, 0) ccw
  line L357 (69.3168, -92.99) -> (68.2317, -90.5528) construction
  spline S86 degree 3 poles (81.6512, -95.2749) (76.2806, -92.5507) (72.8302, -90.2647) (70.7394, -88.6077) knots 1.081688 1.081688 1.081688 1.081688 2 2 2 2
  line L358 (81.6512, -95.2749) -> (76.2806, -92.5507) construction
  line L359 (76.2806, -92.5507) -> (72.8302, -90.2647) construction
  line L360 (72.8302, -90.2647) -> (70.7394, -88.6077) construction
  spline S87 degree 3 poles (71.9758, -102.7799) (70.6729, -96.9005) (69.3168, -92.99) (68.2317, -90.5528) knots 1.081688 1.081688 1.081688 1.081688 2 2 2 2
  line L361 (71.9758, -102.7799) -> (70.6729, -96.9005) construction
  line L362 (70.6729, -96.9005) -> (69.3168, -92.99) construction
  arc A91 (72.9503, -103.9579) -> (82.6228, -96.4493) centre (0, 0) ccw
  line L363 (71.9758, -102.7799) -> (72.9503, -103.9579)
  line L364 (81.6512, -95.2749) -> (82.6228, -96.4493)
  arc A92 (79.043, -81.2871) -> (81.2871, -79.043) centre (0, 0) ccw
  line L365 (80.4249, -83.569) -> (79.043, -81.2871) construction
  spline S88 degree 3 poles (92.9485, -84.29) (87.2788, -82.2605) (83.569, -80.4249) (81.2871, -79.043) knots 1.081688 1.081688 1.081688 1.081688 2 2 2 2
  line L366 (92.9485, -84.29) -> (87.2788, -82.2605) construction
  line L367 (87.2788, -82.2605) -> (83.569, -80.4249) construction
  line L368 (83.569, -80.4249) -> (81.2871, -79.043) construction
  spline S89 degree 3 poles (84.29, -92.9485) (82.2605, -87.2788) (80.4249, -83.569) (79.043, -81.2871) knots 1.081688 1.081688 1.081688 1.081688 2 2 2 2
  line L369 (84.29, -92.9485) -> (82.2605, -87.2788) construction
  line L370 (82.2605, -87.2788) -> (80.4249, -83.569) construction
  arc A93 (85.4045, -93.9951) -> (94.0596, -85.3334) centre (0, 0) ccw
  line L371 (84.29, -92.9485) -> (85.4045, -93.9951)
  line L372 (92.9485, -84.29) -> (94.0596, -85.3334)
  arc A94 (88.6077, -70.7394) -> (90.5528, -68.2317) centre (0, 0) ccw
  line L373 (90.2647, -72.8302) -> (88.6077, -70.7394) construction
  spline S90 degree 3 poles (102.7799, -71.9758) (96.9005, -70.6729) (92.99, -69.3168) (90.5528, -68.2317) knots 1.081688 1.081688 1.081688 1.081688 2 2 2 2
  line L374 (102.7799, -71.9758) -> (96.9005, -70.6729) construction
  line L375 (96.9005, -70.6729) -> (92.99, -69.3168) construction
  line L376 (92.99, -69.3168) -> (90.5528, -68.2317) construction
  spline S91 degree 3 poles (95.2749, -81.6512) (92.5507, -76.2806) (90.2647, -72.8302) (88.6077, -70.7394) knots 1.081688 1.081688 1.081688 1.081688 2 2 2 2
  line L377 (95.2749, -81.6512) -> (92.5507, -76.2806) construction
  line L378 (92.5507, -76.2806) -> (90.2647, -72.8302) construction
  arc A95 (96.5117, -82.5499) -> (104.013, -72.8717) centre (0, 0) ccw
  line L379 (95.2749, -81.6512) -> (96.5117, -82.5499)
  line L380 (102.7799, -71.9758) -> (104.013, -72.8717)
  arc A96 (96.775, -59.0761) -> (98.3905, -56.3444) centre (0, 0) ccw
  line L381 (98.681, -60.9427) -> (96.775, -59.0761) construction
  spline S92 degree 3 poles (110.9904, -58.5265) (104.9941, -57.9708) (100.9444, -57.1155) (98.3905, -56.3444) knots 1.081688 1.081688 1.081688 1.081688 2 2 2 2
  line L382 (110.9904, -58.5265) -> (104.9941, -57.9708) construction
  line L383 (104.9941, -57.9708) -> (100.9444, -57.1155) construction
  line L384 (100.9444, -57.1155) -> (98.3905, -56.3444) construction
  spline S93 degree 3 poles (104.7572, -69.0663) (101.3814, -64.0794) (98.681, -60.9427) (96.775, -59.0761) knots 1.081688 1.081688 1.081688 1.081688 2 2 2 2
  line L385 (104.7572, -69.0663) -> (101.3814, -64.0794) construction
  line L386 (101.3814, -64.0794) -> (98.681, -60.9427) construction
  arc A97 (106.097, -69.8028) -> (112.3261, -59.2608) centre (0, 0) ccw
  line L387 (104.7572, -69.0663) -> (106.097, -69.8028)
  line L388 (110.9904, -58.5265) -> (112.3261, -59.2608)
  arc A98 (103.4161, -46.4812) -> (104.6765, -43.5685) centre (0, 0) ccw
  line L389 (105.541, -48.0941) -> (103.4161, -46.4812) construction
  spline S94 degree 3 poles (117.4505, -44.1542) (111.4318, -44.3544) (107.3069, -44.0134) (104.6765, -43.5685) knots 1.081688 1.081688 1.081688 1.081688 2 2 2 2
  line L390 (117.4505, -44.1542) -> (111.4318, -44.3544) construction
  line L391 (111.4318, -44.3544) -> (107.3069, -44.0134) construction
  line L392 (107.3069, -44.0134) -> (104.6765, -43.5685) construction
  spline S95 degree 3 poles (112.5875, -55.3921) (108.6133, -50.8677) (105.541, -48.0941) (103.4161, -46.4812) knots 1.081688 1.081688 1.081688 1.081688 2 2 2 2
  line L393 (112.5875, -55.3921) -> (108.6133, -50.8677) construction
  line L394 (108.6133, -50.8677) -> (105.541, -48.0941) construction
  arc A99 (114.009, -55.9549) -> (118.8677, -44.7153) centre (0, 0) ccw
  line L395 (112.5875, -55.3921) -> (114.009, -55.9549)
  line L396 (117.4505, -44.1542) -> (118.8677, -44.7153)
  arc A100 (108.4262, -33.1532) -> (109.3117, -30.1055) centre (0, 0) ccw
  line L397 (110.7366, -34.4871) -> (108.4262, -33.1532) construction
  spline S96 degree 3 poles (122.0584, -29.0856) (116.1122, -30.0385) (111.9771, -30.2172) (109.3117, -30.1055) knots 1.081688 1.081688 1.081688 1.081688 2 2 2 2
  line L398 (122.0584, -29.0856) -> (116.1122, -30.0385) construction
  line L399 (116.1122, -30.0385) -> (111.9771, -30.2172) construction
  line L400 (111.9771, -30.2172) -> (109.3117, -30.1055) construction
  spline S97 degree 3 poles (118.6422, -40.8444) (114.1323, -36.8537) (110.7366, -34.4871) (108.4262, -33.1532) knots 1.081688 1.081688 1.081688 1.081688 2 2 2 2
  line L401 (118.6422, -40.8444) -> (114.1323, -36.8537) construction
  line L402 (114.1323, -36.8537) -> (110.7366, -34.4871) construction
  arc A101 (120.123, -41.2246) -> (123.5347, -29.4647) centre (0, 0) ccw
  line L403 (118.6422, -40.8444) -> (120.123, -41.2246)
  line L404 (122.0584, -29.0856) -> (123.5347, -29.4647)
  arc A102 (111.7265, -19.3024) -> (112.2229, -16.1677) centre (0, 0) ccw